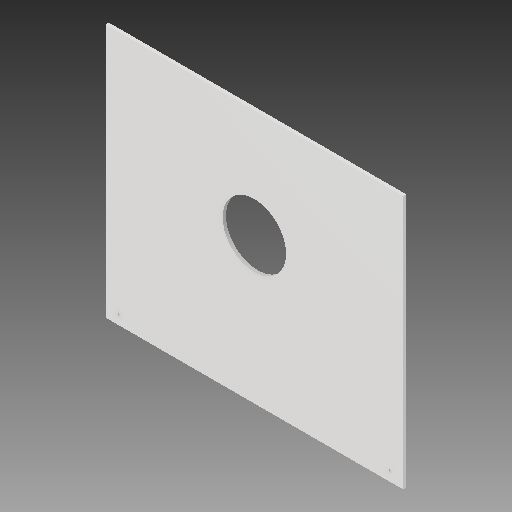
# Autodesk Inventor part: 56.25x48 Gyp
Saved by Autodesk Inventor 2017 (Build 210142000, 142)
## iProperties
Created: 2017-05-25
Part Number: 56.25x48 Gyp
Material: Generic
Document SubType Name: Modeling
Designer: cas7
Density: 1 g/cm^3
Appearance: Default
Mass: 26490.8 g
Surface Area: 34379.7 cm^2
Volume: 26490.8 cm^3
Author: cas7
Autodesk Inventor part; units mm, degrees
ref_plane "YZ Plane" through (0, 0, 0) normal (1, 0, 0) x (0, 1, 0)
ref_plane "XZ Plane" through (0, 0, 0) normal (0, 1, 0) x (-1, 0, 0)
ref_plane "XY Plane" through (0, 0, 0) normal (0, 0, 1) x (1, 0, 0)
sketch "Sketch1" plane through (0, 0, 0) normal (0, 0, 1) x (1, 0, 0)
  line L0 (0, 0) -> (1428.75, 0)
  line L1 (1428.75, 1219.2) -> (0, 1219.2)
  line L2 (0, 1219.2) -> (0, 0)
  line L3 (0, 0) -> (1428.75, 0)
  line L4 (1428.75, 1219.2) -> (0, 1219.2)
  line L5 (0, 1219.2) -> (0, 0)
  line L6 (0, 1219.2) -> (1428.75, 1219.2)
  line L7 (1428.75, 1219.2) -> (1428.75, 0)
  constraints: 16 end point, 3 equal length, 2 horizontal
extrude "Extrusion1" add sketch "Sketch1" along normal blind 15.875
sketch "Sketch2" plane through (0, 0, 15.875) normal (0, 0, 1) x (1, 0, 0)
  circle A0 centre (714.375, 698.5) radius 152.4
  constraints: 1 centre point
extrude "Extrusion2" cut sketch "Sketch2" against normal blind 15.875
sketch "Sketch3" plane through (0, 0, 15.875) normal (0, 0, 1) x (1, 0, 0)
  line L0 (1428.75, 0) -> (1428.75, 1219.2) projected
  line L1 (0, 0) -> (63.5, 0)
  point P0 (1365.25, 44.45)
  point P1 (63.5, 44.45)
  constraints: 2 end point, 1 horizontal
hole "Hole1" at (1365.25, 44.45, 15.875) at (63.5, 44.45, 15.875) direction (0, 0, -1) diameter 12.7 end through all
body "Solid1"
